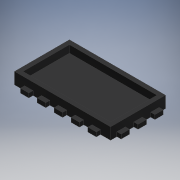
# Autodesk Inventor part: top
Saved by Autodesk Inventor 2019 (Build 230136000, 136)
## iProperties
Created: 2018-06-06
Part Number: top
Material: PBT Plastic Black
Document SubType Name: Modeling
Designer: stra92745
Density: 1.31 g/cm^3
Appearance: Smooth - White
Author: stra92745
Autodesk Inventor part; units mm, degrees
ref_plane "YZ Plane" through (0, 0, 0) normal (1, 0, 0) x (0, 1, 0)
ref_plane "XZ Plane" through (0, 0, 0) normal (0, 1, 0) x (-1, 0, 0)
ref_plane "XY Plane" through (0, 0, 0) normal (0, 0, 1) x (1, 0, 0)
sketch "Sketch1" plane through (0, 0, 0) normal (0, 1, 0) x (-1, 0, 0)
  line L0 (0, 0) -> (-99, 0)
  line L1 (-99, 0) -> (-99, -60)
  line L2 (-99, -60) -> (0, -60)
  line L3 (0, -60) -> (0, 0)
  dimension "d0" = 99
  dimension "d1" = 60
  constraints: 8 end point, 2 parallel, 1 horizontal, 1 perpendicular
  measures "d0" distance of L2.end L1.end
  measures "d1" distance of L1.end L0.end
extrude "Extrusion1" add sketch "Sketch1" along normal blind 4
sketch "Sketch3" plane through (0, 4, 0) normal (0, 1, 0) x (1, 0, 0)
  line L0 (99, 60) -> (0, 60) construction
  line L1 (0, 60) -> (0, 0) construction
  line L2 (0, 0) -> (99, 0) construction
  line L3 (99, 0) -> (99, 60) construction
  line L4 (4, 56) -> (95, 56) construction
  line L5 (95, 56) -> (95, 4) construction
  line L6 (95, 4) -> (4, 4) construction
  line L7 (4, 4) -> (4, 56) construction
  line L8 (0, 30) -> (99, 30) construction
  line L9 (49.5, 0) -> (49.5, 60) construction
  line L10 (0, 50) -> (0, 60)
  line L11 (0, 60) -> (13.5, 60)
  line L12 (13.5, 60) -> (13.5, 56)
  line L13 (13.5, 56) -> (4, 56)
  line L14 (4, 56) -> (4, 50)
  line L15 (4, 50) -> (0, 50)
  line L16 (0, 34) -> (4, 34)
  line L17 (4, 34) -> (4, 42)
  line L18 (4, 42) -> (0, 42)
  line L19 (0, 42) -> (0, 34)
  line L20 (45.5, 56) -> (37.5, 56)
  line L21 (37.5, 56) -> (37.5, 60)
  line L22 (37.5, 60) -> (45.5, 60)
  line L23 (45.5, 60) -> (45.5, 56)
  line L24 (29.5, 56) -> (21.5, 56)
  line L25 (21.5, 56) -> (21.5, 60)
  line L26 (21.5, 60) -> (29.5, 60)
  line L27 (29.5, 60) -> (29.5, 56)
  line L28 (0, 10) -> (0, 0)
  line L29 (0, 0) -> (13.5, 0)
  line L30 (13.5, 0) -> (13.5, 4)
  line L31 (13.5, 4) -> (4, 4)
  line L32 (4, 4) -> (4, 10)
  line L33 (4, 10) -> (0, 10)
  line L34 (0, 26) -> (4, 26)
  line L35 (4, 26) -> (4, 18)
  line L36 (4, 18) -> (0, 18)
  line L37 (0, 18) -> (0, 26)
  line L38 (45.5, 4) -> (37.5, 4)
  line L39 (37.5, 4) -> (37.5, 0)
  line L40 (37.5, 0) -> (45.5, 0)
  line L41 (45.5, 0) -> (45.5, 4)
  line L42 (29.5, 4) -> (21.5, 4)
  line L43 (21.5, 4) -> (21.5, 0)
  line L44 (21.5, 0) -> (29.5, 0)
  line L45 (29.5, 0) -> (29.5, 4)
  line L46 (99, 60) -> (99, 0) construction
  line L47 (95, 4) -> (95, 56) construction
  line L48 (99, 50) -> (99, 60)
  line L49 (99, 60) -> (85.5, 60)
  line L50 (85.5, 60) -> (85.5, 56)
  line L51 (85.5, 56) -> (95, 56)
  line L52 (95, 56) -> (95, 50)
  line L53 (95, 50) -> (99, 50)
  line L54 (99, 34) -> (95, 34)
  line L55 (95, 34) -> (95, 42)
  line L56 (95, 42) -> (99, 42)
  line L57 (99, 42) -> (99, 34)
  line L58 (53.5, 56) -> (61.5, 56)
  line L59 (61.5, 56) -> (61.5, 60)
  line L60 (61.5, 60) -> (53.5, 60)
  line L61 (53.5, 60) -> (53.5, 56)
  line L62 (69.5, 56) -> (77.5, 56)
  line L63 (77.5, 56) -> (77.5, 60)
  line L64 (77.5, 60) -> (69.5, 60)
  line L65 (69.5, 60) -> (69.5, 56)
  line L66 (77.5, 4) -> (77.5, 0)
  line L67 (69.5, 4) -> (77.5, 4)
  line L68 (77.5, 0) -> (69.5, 0)
  line L69 (69.5, 0) -> (69.5, 4)
  line L70 (61.5, 4) -> (61.5, 0)
  line L71 (53.5, 0) -> (53.5, 4)
  line L72 (53.5, 4) -> (61.5, 4)
  line L73 (61.5, 0) -> (53.5, 0)
  line L74 (85.5, 0) -> (85.5, 4)
  line L75 (85.5, 4) -> (95, 4)
  line L76 (95, 4) -> (95, 10)
  line L77 (99, 0) -> (85.5, 0)
  line L78 (99, 10) -> (99, 0)
  line L79 (95, 10) -> (99, 10)
  line L80 (95, 18) -> (99, 18)
  line L81 (95, 26) -> (95, 18)
  line L82 (99, 18) -> (99, 26)
  line L83 (99, 26) -> (95, 26)
  dimension "d11" = 4
  dimension "d12" = 8
  dimension "d13" = 4
  dimension "d14" = 8
  dimension "d15" = 8
  dimension "d16" = 4
  dimension "d17" = 8
  dimension "d18" = 8
  dimension "d19" = 8
  constraints: 160 end point, 48 symmetric about line, 14 point on line, 6 parallel, 5 perpendicular, 4 midpoint, 3 horizontal, 2 collinear, 3 other
  measures "d11" distance between parallel lines of L0 L4
  measures "d12" distance of L16.end L17.end
  measures "d13" distance between parallel lines of L8 L16
  measures "d14" distance between parallel lines of L15 L18
  measures "d15" distance of L20.start L20.end
  measures "d16" distance between parallel lines of L9 L23
  measures "d17" distance of L24.start L24.end
  measures "d18" distance between parallel lines of L21 L27
  measures "d19" distance between parallel lines of L12 L25
extrude "Extrusion3" cut sketch "Sketch3" against normal up to surface (4 mm away)
sketch "Sketch5" plane through (0, 4, 0) normal (0, 1, 0) x (1, 0, 0)
  line L0 (77.5, 0) -> (85.5, 0) projected
  line L1 (99, 42) -> (99, 50) projected
  line L2 (21.5, 60) -> (13.5, 60) projected
  line L3 (0, 18) -> (0, 10) projected
  line L4 (4, 56) -> (95, 56)
  line L5 (95, 56) -> (95, 4)
  line L6 (95, 4) -> (4, 4)
  line L7 (4, 4) -> (4, 56)
  line L8 (91, 52) -> (8, 52)
  line L9 (8, 52) -> (8, 8)
  line L10 (8, 8) -> (91, 8)
  line L11 (91, 8) -> (91, 52)
  line L12 (13.5, 60) -> (13.5, 56) projected
  line L13 (13.5, 56) -> (4, 56) projected
  line L14 (4, 56) -> (4, 50) projected
  line L15 (4, 50) -> (0, 50) projected
  line L16 (0, 50) -> (0, 42) projected
  line L17 (0, 42) -> (4, 42) projected
  line L18 (4, 42) -> (4, 34) projected
  line L19 (4, 34) -> (0, 34) projected
  line L20 (0, 34) -> (0, 26) projected
  line L21 (0, 26) -> (4, 26) projected
  line L22 (4, 26) -> (4, 18) projected
  line L23 (4, 18) -> (0, 18) projected
  line L24 (0, 10) -> (4, 10) projected
  line L25 (4, 10) -> (4, 4) projected
  line L26 (4, 4) -> (13.5, 4) projected
  line L27 (13.5, 4) -> (13.5, 0) projected
  line L28 (13.5, 0) -> (21.5, 0) projected
  line L29 (21.5, 0) -> (21.5, 4) projected
  line L30 (21.5, 4) -> (29.5, 4) projected
  line L31 (29.5, 4) -> (29.5, 0) projected
  line L32 (29.5, 0) -> (37.5, 0) projected
  line L33 (37.5, 0) -> (37.5, 4) projected
  line L34 (37.5, 4) -> (45.5, 4) projected
  line L35 (45.5, 4) -> (45.5, 0) projected
  line L36 (45.5, 0) -> (53.5, 0) projected
  line L37 (53.5, 0) -> (53.5, 4) projected
  line L38 (53.5, 4) -> (61.5, 4) projected
  line L39 (61.5, 4) -> (61.5, 0) projected
  line L40 (61.5, 0) -> (69.5, 0) projected
  line L41 (69.5, 0) -> (69.5, 4) projected
  line L42 (69.5, 4) -> (77.5, 4) projected
  line L43 (77.5, 4) -> (77.5, 0) projected
  line L44 (85.5, 0) -> (85.5, 4) projected
  line L45 (85.5, 4) -> (95, 4) projected
  line L46 (95, 4) -> (95, 10) projected
  line L47 (95, 10) -> (99, 10) projected
  line L48 (99, 10) -> (99, 18) projected
  line L49 (99, 18) -> (95, 18) projected
  line L50 (95, 18) -> (95, 26) projected
  line L51 (95, 26) -> (99, 26) projected
  line L52 (99, 26) -> (99, 34) projected
  line L53 (99, 34) -> (95, 34) projected
  line L54 (95, 34) -> (95, 42) projected
  line L55 (95, 42) -> (99, 42) projected
  line L56 (99, 50) -> (95, 50) projected
  line L57 (95, 50) -> (95, 56) projected
  line L58 (95, 56) -> (85.5, 56) projected
  line L59 (85.5, 56) -> (85.5, 60) projected
  line L60 (85.5, 60) -> (77.5, 60) projected
  line L61 (77.5, 60) -> (77.5, 56) projected
  line L62 (77.5, 56) -> (69.5, 56) projected
  line L63 (69.5, 56) -> (69.5, 60) projected
  line L64 (69.5, 60) -> (61.5, 60) projected
  line L65 (61.5, 60) -> (61.5, 56) projected
  line L66 (61.5, 56) -> (53.5, 56) projected
  line L67 (53.5, 56) -> (53.5, 60) projected
  line L68 (53.5, 60) -> (45.5, 60) projected
  line L69 (45.5, 60) -> (45.5, 56) projected
  line L70 (45.5, 56) -> (37.5, 56) projected
  line L71 (37.5, 56) -> (37.5, 60) projected
  line L72 (37.5, 60) -> (29.5, 60) projected
  line L73 (29.5, 60) -> (29.5, 56) projected
  line L74 (29.5, 56) -> (21.5, 56) projected
  line L75 (21.5, 56) -> (21.5, 60) projected
  point P0 (0, 0)
  dimension "d22" = 4
  dimension "d23" = 4
  constraints: 16 end point, 6 other
  measures "d22" distance between parallel lines of L2 L4
  measures "d23" distance between parallel lines of L4 L8
extrude "Extrusion4" add sketch "Sketch5" along normal blind 7 contours L6 L7 L4 L5
body "Solid1"
